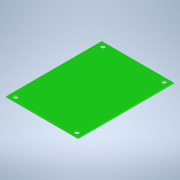
# Autodesk Inventor part: Mock Module PCB
Saved by Autodesk Inventor 2022 (Build 260153000, 153)
## iProperties
Created: 2021-07-19
Part Number: Mock Module PCB
Material: Generic
Document SubType Name: Modeling
Designer: Caleb
Density: 1 g/cm^3
Appearance: Dark Green
Author: Caleb
Autodesk Inventor part; units mm, degrees
(part 1 of 2)
ref_plane "YZ Plane" through (0, 0, 0) normal (1, 0, 0) x (0, 1, 0)
ref_plane "XZ Plane" through (0, 0, 0) normal (0, 1, 0) x (-1, 0, 0)
ref_plane "XY Plane" through (0, 0, 0) normal (0, 0, 1) x (1, 0, 0)
sketch "Sketch1" plane through (0, 0, 0) normal (0, 1, 0) x (-1, 0, 0)
  line L0 (-21.3, 28.25) -> (21.3, 28.25)
  line L1 (21.3, 28.25) -> (21.3, -28.25)
  line L2 (21.3, -28.25) -> (-21.3, -28.25)
  line L3 (-21.3, -28.25) -> (-21.3, 28.25)
  line L4 (-21.3, 28.25) -> (21.3, -28.25) construction
  line L5 (21.3, 28.25) -> (-21.3, -28.25) construction
  point P0 (0, 0)
  dimension "d0" = 42.6
  dimension "d1" = 56.5
  constraints: 12 end point, 2 midpoint, 2 parallel, 1 horizontal, 1 perpendicular
  measures "d0" distance of L0.start L0.end
  measures "d1" distance of L0.end L1.end
extrude "Extrusion1" add sketch "Sketch1" along normal blind 0.5
sketch "Sketch6" plane through (0, 0.5, 0) normal (0, 1, 0) x (1, 0, 0)
  point P0 (0, 0)
  point P1 (-18.05, -25.75)
  point P2 (18.05, -25.75)
  point P3 (18.05, 25.75)
  point P4 (-18.05, 25.75)
  dimension "d33" = 51.5
  dimension "d34" = 36.1
  dimension "d35" = 25.75
  dimension "d36" = 18.05
  constraints: 2 horizontal alignment, 2 vertical alignment
  measures "d33" distance of point (-18.05, -25.75) point (-18.05, 25.75)
  measures "d34" distance of point (18.05, -25.75) point (-18.05, -25.75)
  measures "d35" vertical distance of point (-18.05, -25.75) point (0, 0)
  measures "d36" horizontal distance of point (-18.05, -25.75) point (0, 0)
hole "Hole2" at (-18.05, 0.5, -25.75) at (18.05, 0.5, -25.75) at (18.05, 0.5, 25.75) at (-18.05, 0.5, 25.75) direction (0, -1, 0) diameter 2.2 end through all clearance for "Flat Head Machine Screw" size "M2" standard "Ansi Metric M Profile"
sketch "Sketch7" plane through (0, 0, 0) normal (0, -1, 0) x (1, 0, 0)
  line L0 (-18.3, -24.35) -> (-18.22, -24.35)
  line L1 (-18.22, -24.35) -> (-18.22, -24.05)
  line L2 (-18.22, -24.05) -> (-18.3, -24.05)
  line L3 (-18.3, -24.05) -> (-18.3, -24.35)
  line L4 (-21.3, -28.25) -> (-21.3, 28.25) projected
  line L5 (21.3, -28.25) -> (-21.3, -28.25) projected
  line L6 (-18.175, -24.35) -> (-18.095, -24.35)
  line L7 (-18.095, -24.35) -> (-18.095, -24.05)
  line L8 (-18.095, -24.05) -> (-18.175, -24.05)
  line L9 (-18.175, -24.05) -> (-18.175, -24.35)
  line L10 (-18.05, -24.35) -> (-17.97, -24.35)
  line L11 (-17.97, -24.35) -> (-17.97, -24.05)
  line L12 (-17.97, -24.05) -> (-18.05, -24.05)
  line L13 (-18.05, -24.05) -> (-18.05, -24.35)
  line L14 (-17.925, -24.35) -> (-17.845, -24.35)
  line L15 (-17.845, -24.35) -> (-17.845, -24.05)
  line L16 (-17.845, -24.05) -> (-17.925, -24.05)
  line L17 (-17.925, -24.05) -> (-17.925, -24.35)
  line L18 (-17.8, -24.35) -> (-17.72, -24.35)
  line L19 (-17.72, -24.35) -> (-17.72, -24.05)
  line L20 (-17.72, -24.05) -> (-17.8, -24.05)
  line L21 (-17.8, -24.05) -> (-17.8, -24.35)
  line L22 (-17.675, -24.35) -> (-17.595, -24.35)
  line L23 (-17.595, -24.35) -> (-17.595, -24.05)
  line L24 (-17.595, -24.05) -> (-17.675, -24.05)
  line L25 (-17.675, -24.05) -> (-17.675, -24.35)
  line L26 (-17.55, -24.35) -> (-17.47, -24.35)
  line L27 (-17.47, -24.35) -> (-17.47, -24.05)
  line L28 (-17.47, -24.05) -> (-17.55, -24.05)
  line L29 (-17.55, -24.05) -> (-17.55, -24.35)
  line L30 (-17.425, -24.35) -> (-17.345, -24.35)
  line L31 (-17.345, -24.35) -> (-17.345, -24.05)
  line L32 (-17.345, -24.05) -> (-17.425, -24.05)
  line L33 (-17.425, -24.05) -> (-17.425, -24.35)
  line L34 (-17.3, -24.35) -> (-17.22, -24.35)
  line L35 (-17.22, -24.35) -> (-17.22, -24.05)
  line L36 (-17.22, -24.05) -> (-17.3, -24.05)
  line L37 (-17.3, -24.05) -> (-17.3, -24.35)
  line L38 (-17.175, -24.35) -> (-17.095, -24.35)
  line L39 (-17.095, -24.35) -> (-17.095, -24.05)
  line L40 (-17.095, -24.05) -> (-17.175, -24.05)
  line L41 (-17.175, -24.05) -> (-17.175, -24.35)
  line L42 (-17.05, -24.35) -> (-16.97, -24.35)
  line L43 (-16.97, -24.35) -> (-16.97, -24.05)
  line L44 (-16.97, -24.05) -> (-17.05, -24.05)
  line L45 (-17.05, -24.05) -> (-17.05, -24.35)
  line L46 (-16.925, -24.35) -> (-16.845, -24.35)
  line L47 (-16.845, -24.35) -> (-16.845, -24.05)
  line L48 (-16.845, -24.05) -> (-16.925, -24.05)
  line L49 (-16.925, -24.05) -> (-16.925, -24.35)
  line L50 (-16.8, -24.35) -> (-16.72, -24.35)
  line L51 (-16.72, -24.35) -> (-16.72, -24.05)
  line L52 (-16.72, -24.05) -> (-16.8, -24.05)
  line L53 (-16.8, -24.05) -> (-16.8, -24.35)
  line L54 (-16.675, -24.35) -> (-16.595, -24.35)
  line L55 (-16.595, -24.35) -> (-16.595, -24.05)
  line L56 (-16.595, -24.05) -> (-16.675, -24.05)
  line L57 (-16.675, -24.05) -> (-16.675, -24.35)
  line L58 (-16.55, -24.35) -> (-16.47, -24.35)
  line L59 (-16.47, -24.35) -> (-16.47, -24.05)
  line L60 (-16.47, -24.05) -> (-16.55, -24.05)
  line L61 (-16.55, -24.05) -> (-16.55, -24.35)
  line L62 (-16.425, -24.35) -> (-16.345, -24.35)
  line L63 (-16.345, -24.35) -> (-16.345, -24.05)
  line L64 (-16.345, -24.05) -> (-16.425, -24.05)
  line L65 (-16.425, -24.05) -> (-16.425, -24.35)
  line L66 (-16.3, -24.35) -> (-16.22, -24.35)
  line L67 (-16.22, -24.35) -> (-16.22, -24.05)
  line L68 (-16.22, -24.05) -> (-16.3, -24.05)
  line L69 (-16.3, -24.05) -> (-16.3, -24.35)
  line L70 (-16.175, -24.35) -> (-16.095, -24.35)
  line L71 (-16.095, -24.35) -> (-16.095, -24.05)
  line L72 (-16.095, -24.05) -> (-16.175, -24.05)
  line L73 (-16.175, -24.05) -> (-16.175, -24.35)
  line L74 (-16.05, -24.35) -> (-15.97, -24.35)
  line L75 (-15.97, -24.35) -> (-15.97, -24.05)
  line L76 (-15.97, -24.05) -> (-16.05, -24.05)
  line L77 (-16.05, -24.05) -> (-16.05, -24.35)
  line L78 (-15.925, -24.35) -> (-15.845, -24.35)
  line L79 (-15.845, -24.35) -> (-15.845, -24.05)
  line L80 (-15.845, -24.05) -> (-15.925, -24.05)
  line L81 (-15.925, -24.05) -> (-15.925, -24.35)
  line L82 (-15.8, -24.35) -> (-15.72, -24.35)
  line L83 (-15.72, -24.35) -> (-15.72, -24.05)
  line L84 (-15.72, -24.05) -> (-15.8, -24.05)
  line L85 (-15.8, -24.05) -> (-15.8, -24.35)
  line L86 (-15.675, -24.35) -> (-15.595, -24.35)
  line L87 (-15.595, -24.35) -> (-15.595, -24.05)
  line L88 (-15.595, -24.05) -> (-15.675, -24.05)
  line L89 (-15.675, -24.05) -> (-15.675, -24.35)
  line L90 (-15.55, -24.35) -> (-15.47, -24.35)
  line L91 (-15.47, -24.35) -> (-15.47, -24.05)
  line L92 (-15.47, -24.05) -> (-15.55, -24.05)
  line L93 (-15.55, -24.05) -> (-15.55, -24.35)
  line L94 (-15.425, -24.35) -> (-15.345, -24.35)
  line L95 (-15.345, -24.35) -> (-15.345, -24.05)
  line L96 (-15.345, -24.05) -> (-15.425, -24.05)
  line L97 (-15.425, -24.05) -> (-15.425, -24.35)
  line L98 (-15.3, -24.35) -> (-15.22, -24.35)
  line L99 (-15.22, -24.35) -> (-15.22, -24.05)
  line L100 (-15.22, -24.05) -> (-15.3, -24.05)
  line L101 (-15.3, -24.05) -> (-15.3, -24.35)
  line L102 (-15.175, -24.35) -> (-15.095, -24.35)
  line L103 (-15.095, -24.35) -> (-15.095, -24.05)
  line L104 (-15.095, -24.05) -> (-15.175, -24.05)
  line L105 (-15.175, -24.05) -> (-15.175, -24.35)
  line L106 (-15.05, -24.35) -> (-14.97, -24.35)
  line L107 (-14.97, -24.35) -> (-14.97, -24.05)
  line L108 (-14.97, -24.05) -> (-15.05, -24.05)
  line L109 (-15.05, -24.05) -> (-15.05, -24.35)
  line L110 (-14.925, -24.35) -> (-14.845, -24.35)
  line L111 (-14.845, -24.35) -> (-14.845, -24.05)
  line L112 (-14.845, -24.05) -> (-14.925, -24.05)
  line L113 (-14.925, -24.05) -> (-14.925, -24.35)
  line L114 (-14.8, -24.35) -> (-14.72, -24.35)
  line L115 (-14.72, -24.35) -> (-14.72, -24.05)
  line L116 (-14.72, -24.05) -> (-14.8, -24.05)
  line L117 (-14.8, -24.05) -> (-14.8, -24.35)
  line L118 (-14.675, -24.35) -> (-14.595, -24.35)
  line L119 (-14.595, -24.35) -> (-14.595, -24.05)
  line L120 (-14.595, -24.05) -> (-14.675, -24.05)
  line L121 (-14.675, -24.05) -> (-14.675, -24.35)
  line L122 (-14.55, -24.35) -> (-14.47, -24.35)
  line L123 (-14.47, -24.35) -> (-14.47, -24.05)
  line L124 (-14.47, -24.05) -> (-14.55, -24.05)
  line L125 (-14.55, -24.05) -> (-14.55, -24.35)
  line L126 (-14.425, -24.35) -> (-14.345, -24.35)
  line L127 (-14.345, -24.35) -> (-14.345, -24.05)
  line L128 (-14.345, -24.05) -> (-14.425, -24.05)
  line L129 (-14.425, -24.05) -> (-14.425, -24.35)
  line L130 (-14.3, -24.35) -> (-14.22, -24.35)
  line L131 (-14.22, -24.35) -> (-14.22, -24.05)
  line L132 (-14.22, -24.05) -> (-14.3, -24.05)
  line L133 (-14.3, -24.05) -> (-14.3, -24.35)
  line L134 (-14.175, -24.35) -> (-14.095, -24.35)
  line L135 (-14.095, -24.35) -> (-14.095, -24.05)
  line L136 (-14.095, -24.05) -> (-14.175, -24.05)
  line L137 (-14.175, -24.05) -> (-14.175, -24.35)
  line L138 (-14.05, -24.35) -> (-13.97, -24.35)
  line L139 (-13.97, -24.35) -> (-13.97, -24.05)
  line L140 (-13.97, -24.05) -> (-14.05, -24.05)
  line L141 (-14.05, -24.05) -> (-14.05, -24.35)
  line L142 (-13.925, -24.35) -> (-13.845, -24.35)
  line L143 (-13.845, -24.35) -> (-13.845, -24.05)
  line L144 (-13.845, -24.05) -> (-13.925, -24.05)
  line L145 (-13.925, -24.05) -> (-13.925, -24.35)
  line L146 (-13.8, -24.35) -> (-13.72, -24.35)
  line L147 (-13.72, -24.35) -> (-13.72, -24.05)
  line L148 (-13.72, -24.05) -> (-13.8, -24.05)
  line L149 (-13.8, -24.05) -> (-13.8, -24.35)
  line L150 (-13.675, -24.35) -> (-13.595, -24.35)
  line L151 (-13.595, -24.35) -> (-13.595, -24.05)
  line L152 (-13.595, -24.05) -> (-13.675, -24.05)
  line L153 (-13.675, -24.05) -> (-13.675, -24.35)
  line L154 (-13.55, -24.35) -> (-13.47, -24.35)
  line L155 (-13.47, -24.35) -> (-13.47, -24.05)
  line L156 (-13.47, -24.05) -> (-13.55, -24.05)
  line L157 (-13.55, -24.05) -> (-13.55, -24.35)
  line L158 (-13.425, -24.35) -> (-13.345, -24.35)
  line L159 (-13.345, -24.35) -> (-13.345, -24.05)
  line L160 (-13.345, -24.05) -> (-13.425, -24.05)
  line L161 (-13.425, -24.05) -> (-13.425, -24.35)
  line L162 (-13.3, -24.35) -> (-13.22, -24.35)
  line L163 (-13.22, -24.35) -> (-13.22, -24.05)
  line L164 (-13.22, -24.05) -> (-13.3, -24.05)
  line L165 (-13.3, -24.05) -> (-13.3, -24.35)
  line L166 (-13.175, -24.35) -> (-13.095, -24.35)
  line L167 (-13.095, -24.35) -> (-13.095, -24.05)
  line L168 (-13.095, -24.05) -> (-13.175, -24.05)
  line L169 (-13.175, -24.05) -> (-13.175, -24.35)
  line L170 (-13.05, -24.35) -> (-12.97, -24.35)
  line L171 (-12.97, -24.35) -> (-12.97, -24.05)
  line L172 (-12.97, -24.05) -> (-13.05, -24.05)
  line L173 (-13.05, -24.05) -> (-13.05, -24.35)
  line L174 (-12.925, -24.35) -> (-12.845, -24.35)
  line L175 (-12.845, -24.35) -> (-12.845, -24.05)
  line L176 (-12.845, -24.05) -> (-12.925, -24.05)
  line L177 (-12.925, -24.05) -> (-12.925, -24.35)
  line L178 (-12.8, -24.35) -> (-12.72, -24.35)
  line L179 (-12.72, -24.35) -> (-12.72, -24.05)
  line L180 (-12.72, -24.05) -> (-12.8, -24.05)
  line L181 (-12.8, -24.05) -> (-12.8, -24.35)
  line L182 (-12.675, -24.35) -> (-12.595, -24.35)
  line L183 (-12.595, -24.35) -> (-12.595, -24.05)
  line L184 (-12.595, -24.05) -> (-12.675, -24.05)
  line L185 (-12.675, -24.05) -> (-12.675, -24.35)
  line L186 (-12.55, -24.35) -> (-12.47, -24.35)
  line L187 (-12.47, -24.35) -> (-12.47, -24.05)
  line L188 (-12.47, -24.05) -> (-12.55, -24.05)
  line L189 (-12.55, -24.05) -> (-12.55, -24.35)
  line L190 (-12.425, -24.35) -> (-12.345, -24.35)
  line L191 (-12.345, -24.35) -> (-12.345, -24.05)
  line L192 (-12.345, -24.05) -> (-12.425, -24.05)
  line L193 (-12.425, -24.05) -> (-12.425, -24.35)
  line L194 (-12.3, -24.35) -> (-12.22, -24.35)
  line L195 (-12.22, -24.35) -> (-12.22, -24.05)
  line L196 (-12.22, -24.05) -> (-12.3, -24.05)
  line L197 (-12.3, -24.05) -> (-12.3, -24.35)
  line L198 (-12.175, -24.35) -> (-12.095, -24.35)
  line L199 (-12.095, -24.35) -> (-12.095, -24.05)
  line L200 (-12.095, -24.05) -> (-12.175, -24.05)
  line L201 (-12.175, -24.05) -> (-12.175, -24.35)
  line L202 (-12.05, -24.35) -> (-11.97, -24.35)
  line L203 (-11.97, -24.35) -> (-11.97, -24.05)
  line L204 (-11.97, -24.05) -> (-12.05, -24.05)
  line L205 (-12.05, -24.05) -> (-12.05, -24.35)
  line L206 (-11.925, -24.35) -> (-11.845, -24.35)
  line L207 (-11.845, -24.35) -> (-11.845, -24.05)
  line L208 (-11.845, -24.05) -> (-11.925, -24.05)
  line L209 (-11.925, -24.05) -> (-11.925, -24.35)
  line L210 (-11.8, -24.35) -> (-11.72, -24.35)
  line L211 (-11.72, -24.35) -> (-11.72, -24.05)
  line L212 (-11.72, -24.05) -> (-11.8, -24.05)
  line L213 (-11.8, -24.05) -> (-11.8, -24.35)
  line L214 (-11.675, -24.35) -> (-11.595, -24.35)
  line L215 (-11.595, -24.35) -> (-11.595, -24.05)
  line L216 (-11.595, -24.05) -> (-11.675, -24.05)
  line L217 (-11.675, -24.05) -> (-11.675, -24.35)
  line L218 (-11.55, -24.35) -> (-11.47, -24.35)
  line L219 (-11.47, -24.35) -> (-11.47, -24.05)
  line L220 (-11.47, -24.05) -> (-11.55, -24.05)
  line L221 (-11.55, -24.05) -> (-11.55, -24.35)
  line L222 (-11.425, -24.35) -> (-11.345, -24.35)
  line L223 (-11.345, -24.35) -> (-11.345, -24.05)
  line L224 (-11.345, -24.05) -> (-11.425, -24.05)
  line L225 (-11.425, -24.05) -> (-11.425, -24.35)
  line L226 (-11.3, -24.35) -> (-11.22, -24.35)
  line L227 (-11.22, -24.35) -> (-11.22, -24.05)
  line L228 (-11.22, -24.05) -> (-11.3, -24.05)
  line L229 (-11.3, -24.05) -> (-11.3, -24.35)
  line L230 (-11.175, -24.35) -> (-11.095, -24.35)
  line L231 (-11.095, -24.35) -> (-11.095, -24.05)
  line L232 (-11.095, -24.05) -> (-11.175, -24.05)
  line L233 (-11.175, -24.05) -> (-11.175, -24.35)
  line L234 (-11.05, -24.35) -> (-10.97, -24.35)
  line L235 (-10.97, -24.35) -> (-10.97, -24.05)
  line L236 (-10.97, -24.05) -> (-11.05, -24.05)
  line L237 (-11.05, -24.05) -> (-11.05, -24.35)
  line L238 (-10.925, -24.35) -> (-10.845, -24.35)
  line L239 (-10.845, -24.35) -> (-10.845, -24.05)
  line L240 (-10.845, -24.05) -> (-10.925, -24.05)
  line L241 (-10.925, -24.05) -> (-10.925, -24.35)
  line L242 (-10.8, -24.35) -> (-10.72, -24.35)
  line L243 (-10.72, -24.35) -> (-10.72, -24.05)
  line L244 (-10.72, -24.05) -> (-10.8, -24.05)
  line L245 (-10.8, -24.05) -> (-10.8, -24.35)
  line L246 (-10.675, -24.35) -> (-10.595, -24.35)
  line L247 (-10.595, -24.35) -> (-10.595, -24.05)
  line L248 (-10.595, -24.05) -> (-10.675, -24.05)
  line L249 (-10.675, -24.05) -> (-10.675, -24.35)
  line L250 (-10.55, -24.35) -> (-10.47, -24.35)
  line L251 (-10.47, -24.35) -> (-10.47, -24.05)
  line L252 (-10.47, -24.05) -> (-10.55, -24.05)
  line L253 (-10.55, -24.05) -> (-10.55, -24.35)
  line L254 (-10.425, -24.35) -> (-10.345, -24.35)
  line L255 (-10.345, -24.35) -> (-10.345, -24.05)
  line L256 (-10.345, -24.05) -> (-10.425, -24.05)
  line L257 (-10.425, -24.05) -> (-10.425, -24.35)
  line L258 (-10.3, -24.35) -> (-10.22, -24.35)
  line L259 (-10.22, -24.35) -> (-10.22, -24.05)
  line L260 (-10.22, -24.05) -> (-10.3, -24.05)
  line L261 (-10.3, -24.05) -> (-10.3, -24.35)
  line L262 (-10.175, -24.35) -> (-10.095, -24.35)
  line L263 (-10.095, -24.35) -> (-10.095, -24.05)
  line L264 (-10.095, -24.05) -> (-10.175, -24.05)
  line L265 (-10.175, -24.05) -> (-10.175, -24.35)
  line L266 (-10.05, -24.35) -> (-9.97, -24.35)
  line L267 (-9.97, -24.35) -> (-9.97, -24.05)
  line L268 (-9.97, -24.05) -> (-10.05, -24.05)
  line L269 (-10.05, -24.05) -> (-10.05, -24.35)
  line L270 (-9.925, -24.35) -> (-9.845, -24.35)
  line L271 (-9.845, -24.35) -> (-9.845, -24.05)
  line L272 (-9.845, -24.05) -> (-9.925, -24.05)
  line L273 (-9.925, -24.05) -> (-9.925, -24.35)
  line L274 (-9.8, -24.35) -> (-9.72, -24.35)
  line L275 (-9.72, -24.35) -> (-9.72, -24.05)
  line L276 (-9.72, -24.05) -> (-9.8, -24.05)
  line L277 (-9.8, -24.05) -> (-9.8, -24.35)
  line L278 (-9.675, -24.35) -> (-9.595, -24.35)
  line L279 (-9.595, -24.35) -> (-9.595, -24.05)
  line L280 (-9.595, -24.05) -> (-9.675, -24.05)
  line L281 (-9.675, -24.05) -> (-9.675, -24.35)
  line L282 (-9.55, -24.35) -> (-9.47, -24.35)
  line L283 (-9.47, -24.35) -> (-9.47, -24.05)
  line L284 (-9.47, -24.05) -> (-9.55, -24.05)
  line L285 (-9.55, -24.05) -> (-9.55, -24.35)
  line L286 (-9.425, -24.35) -> (-9.345, -24.35)
  line L287 (-9.345, -24.35) -> (-9.345, -24.05)
  line L288 (-9.345, -24.05) -> (-9.425, -24.05)
  line L289 (-9.425, -24.05) -> (-9.425, -24.35)
  line L290 (-9.3, -24.35) -> (-9.22, -24.35)
  line L291 (-9.22, -24.35) -> (-9.22, -24.05)
  line L292 (-9.22, -24.05) -> (-9.3, -24.05)
  line L293 (-9.3, -24.05) -> (-9.3, -24.35)
  line L294 (-9.175, -24.35) -> (-9.095, -24.35)
  line L295 (-9.095, -24.35) -> (-9.095, -24.05)
  line L296 (-9.095, -24.05) -> (-9.175, -24.05)
  line L297 (-9.175, -24.05) -> (-9.175, -24.35)
  line L298 (-9.05, -24.35) -> (-8.97, -24.35)
  line L299 (-8.97, -24.35) -> (-8.97, -24.05)
  line L300 (-8.97, -24.05) -> (-9.05, -24.05)
  line L301 (-9.05, -24.05) -> (-9.05, -24.35)
  line L302 (-8.925, -24.35) -> (-8.845, -24.35)
  line L303 (-8.845, -24.35) -> (-8.845, -24.05)
  line L304 (-8.845, -24.05) -> (-8.925, -24.05)
  line L305 (-8.925, -24.05) -> (-8.925, -24.35)
  line L306 (-8.8, -24.35) -> (-8.72, -24.35)
  line L307 (-8.72, -24.35) -> (-8.72, -24.05)
  line L308 (-8.72, -24.05) -> (-8.8, -24.05)
  line L309 (-8.8, -24.05) -> (-8.8, -24.35)
  line L310 (-8.675, -24.35) -> (-8.595, -24.35)
  line L311 (-8.595, -24.35) -> (-8.595, -24.05)
  line L312 (-8.595, -24.05) -> (-8.675, -24.05)
  line L313 (-8.675, -24.05) -> (-8.675, -24.35)
  line L314 (-8.55, -24.35) -> (-8.47, -24.35)
  line L315 (-8.47, -24.35) -> (-8.47, -24.05)
  line L316 (-8.47, -24.05) -> (-8.55, -24.05)
  line L317 (-8.55, -24.05) -> (-8.55, -24.35)
  line L318 (-8.425, -24.35) -> (-8.345, -24.35)
  line L319 (-8.345, -24.35) -> (-8.345, -24.05)
  line L320 (-8.345, -24.05) -> (-8.425, -24.05)
  line L321 (-8.425, -24.05) -> (-8.425, -24.35)
  line L322 (-8.3, -24.35) -> (-8.22, -24.35)
  line L323 (-8.22, -24.35) -> (-8.22, -24.05)
  line L324 (-8.22, -24.05) -> (-8.3, -24.05)
  line L325 (-8.3, -24.05) -> (-8.3, -24.35)
  line L326 (-8.175, -24.35) -> (-8.095, -24.35)
  line L327 (-8.095, -24.35) -> (-8.095, -24.05)
  line L328 (-8.095, -24.05) -> (-8.175, -24.05)
  line L329 (-8.175, -24.05) -> (-8.175, -24.35)
  line L330 (-8.05, -24.35) -> (-7.97, -24.35)
  line L331 (-7.97, -24.35) -> (-7.97, -24.05)
  line L332 (-7.97, -24.05) -> (-8.05, -24.05)
  line L333 (-8.05, -24.05) -> (-8.05, -24.35)
  line L334 (-7.925, -24.35) -> (-7.845, -24.35)
  line L335 (-7.845, -24.35) -> (-7.845, -24.05)
  line L336 (-7.845, -24.05) -> (-7.925, -24.05)
  line L337 (-7.925, -24.05) -> (-7.925, -24.35)
  line L338 (-7.8, -24.35) -> (-7.72, -24.35)
  line L339 (-7.72, -24.35) -> (-7.72, -24.05)
  line L340 (-7.72, -24.05) -> (-7.8, -24.05)
  line L341 (-7.8, -24.05) -> (-7.8, -24.35)
  line L342 (-7.675, -24.35) -> (-7.595, -24.35)
  line L343 (-7.595, -24.35) -> (-7.595, -24.05)
  line L344 (-7.595, -24.05) -> (-7.675, -24.05)
  line L345 (-7.675, -24.05) -> (-7.675, -24.35)
  line L346 (-7.55, -24.35) -> (-7.47, -24.35)
  line L347 (-7.47, -24.35) -> (-7.47, -24.05)
  line L348 (-7.47, -24.05) -> (-7.55, -24.05)
  line L349 (-7.55, -24.05) -> (-7.55, -24.35)
  line L350 (-7.425, -24.35) -> (-7.345, -24.35)
  line L351 (-7.345, -24.35) -> (-7.345, -24.05)
  line L352 (-7.345, -24.05) -> (-7.425, -24.05)
  line L353 (-7.425, -24.05) -> (-7.425, -24.35)
  line L354 (-7.3, -24.35) -> (-7.22, -24.35)
  line L355 (-7.22, -24.35) -> (-7.22, -24.05)
  line L356 (-7.22, -24.05) -> (-7.3, -24.05)
  line L357 (-7.3, -24.05) -> (-7.3, -24.35)
  line L358 (-7.175, -24.35) -> (-7.095, -24.35)
  line L359 (-7.095, -24.35) -> (-7.095, -24.05)
  line L360 (-7.095, -24.05) -> (-7.175, -24.05)
  line L361 (-7.175, -24.05) -> (-7.175, -24.35)
  line L362 (-7.05, -24.35) -> (-6.97, -24.35)
  line L363 (-6.97, -24.35) -> (-6.97, -24.05)
  line L364 (-6.97, -24.05) -> (-7.05, -24.05)
  line L365 (-7.05, -24.05) -> (-7.05, -24.35)
  line L366 (-6.925, -24.35) -> (-6.845, -24.35)
  line L367 (-6.845, -24.35) -> (-6.845, -24.05)
  line L368 (-6.845, -24.05) -> (-6.925, -24.05)
  line L369 (-6.925, -24.05) -> (-6.925, -24.35)
  line L370 (-6.8, -24.35) -> (-6.72, -24.35)
  line L371 (-6.72, -24.35) -> (-6.72, -24.05)
  line L372 (-6.72, -24.05) -> (-6.8, -24.05)
  line L373 (-6.8, -24.05) -> (-6.8, -24.35)
  line L374 (-6.675, -24.35) -> (-6.595, -24.35)
  line L375 (-6.595, -24.35) -> (-6.595, -24.05)
  line L376 (-6.595, -24.05) -> (-6.675, -24.05)
  line L377 (-6.675, -24.05) -> (-6.675, -24.35)
  line L378 (-6.55, -24.35) -> (-6.47, -24.35)
  line L379 (-6.47, -24.35) -> (-6.47, -24.05)
  line L380 (-6.47, -24.05) -> (-6.55, -24.05)
  line L381 (-6.55, -24.05) -> (-6.55, -24.35)
  line L382 (-6.425, -24.35) -> (-6.345, -24.35)
  line L383 (-6.345, -24.35) -> (-6.345, -24.05)
  line L384 (-6.345, -24.05) -> (-6.425, -24.05)
  line L385 (-6.425, -24.05) -> (-6.425, -24.35)
  line L386 (-6.3, -24.35) -> (-6.22, -24.35)
  line L387 (-6.22, -24.35) -> (-6.22, -24.05)
  line L388 (-6.22, -24.05) -> (-6.3, -24.05)
  line L389 (-6.3, -24.05) -> (-6.3, -24.35)
  line L390 (-6.175, -24.35) -> (-6.095, -24.35)
  line L391 (-6.095, -24.35) -> (-6.095, -24.05)
  line L392 (-6.095, -24.05) -> (-6.175, -24.05)
  line L393 (-6.175, -24.05) -> (-6.175, -24.35)
  line L394 (-6.05, -24.35) -> (-5.97, -24.35)
  line L395 (-5.97, -24.35) -> (-5.97, -24.05)
  line L396 (-5.97, -24.05) -> (-6.05, -24.05)
  line L397 (-6.05, -24.05) -> (-6.05, -24.35)
  line L398 (-5.925, -24.35) -> (-5.845, -24.35)
  line L399 (-5.845, -24.35) -> (-5.845, -24.05)
  line L400 (-5.845, -24.05) -> (-5.925, -24.05)
  line L401 (-5.925, -24.05) -> (-5.925, -24.35)
  line L402 (-5.8, -24.35) -> (-5.72, -24.35)
  line L403 (-5.72, -24.35) -> (-5.72, -24.05)
  line L404 (-5.72, -24.05) -> (-5.8, -24.05)
  line L405 (-5.8, -24.05) -> (-5.8, -24.35)
  line L406 (-5.675, -24.35) -> (-5.595, -24.35)
  line L407 (-5.595, -24.35) -> (-5.595, -24.05)
  line L408 (-5.595, -24.05) -> (-5.675, -24.05)
  line L409 (-5.675, -24.05) -> (-5.675, -24.35)
  line L410 (-5.55, -24.35) -> (-5.47, -24.35)
  line L411 (-5.47, -24.35) -> (-5.47, -24.05)
  line L412 (-5.47, -24.05) -> (-5.55, -24.05)
  line L413 (-5.55, -24.05) -> (-5.55, -24.35)
  line L414 (-5.425, -24.35) -> (-5.345, -24.35)
  line L415 (-5.345, -24.35) -> (-5.345, -24.05)
  line L416 (-5.345, -24.05) -> (-5.425, -24.05)
  line L417 (-5.425, -24.05) -> (-5.425, -24.35)
  line L418 (-5.3, -24.35) -> (-5.22, -24.35)
  line L419 (-5.22, -24.35) -> (-5.22, -24.05)
  line L420 (-5.22, -24.05) -> (-5.3, -24.05)
  line L421 (-5.3, -24.05) -> (-5.3, -24.35)
  line L422 (-5.175, -24.35) -> (-5.095, -24.35)
  line L423 (-5.095, -24.35) -> (-5.095, -24.05)
  line L424 (-5.095, -24.05) -> (-5.175, -24.05)
  line L425 (-5.175, -24.05) -> (-5.175, -24.35)
  line L426 (-5.05, -24.35) -> (-4.97, -24.35)
  line L427 (-4.97, -24.35) -> (-4.97, -24.05)
  line L428 (-4.97, -24.05) -> (-5.05, -24.05)
  line L429 (-5.05, -24.05) -> (-5.05, -24.35)
  line L430 (-4.925, -24.35) -> (-4.845, -24.35)
  line L431 (-4.845, -24.35) -> (-4.845, -24.05)
  line L432 (-4.845, -24.05) -> (-4.925, -24.05)
  line L433 (-4.925, -24.05) -> (-4.925, -24.35)
  line L434 (-4.8, -24.35) -> (-4.72, -24.35)
  line L435 (-4.72, -24.35) -> (-4.72, -24.05)
  line L436 (-4.72, -24.05) -> (-4.8, -24.05)
  line L437 (-4.8, -24.05) -> (-4.8, -24.35)
  line L438 (-4.675, -24.35) -> (-4.595, -24.35)
  line L439 (-4.595, -24.35) -> (-4.595, -24.05)
  line L440 (-4.595, -24.05) -> (-4.675, -24.05)
  line L441 (-4.675, -24.05) -> (-4.675, -24.35)
  line L442 (-4.55, -24.35) -> (-4.47, -24.35)
  line L443 (-4.47, -24.35) -> (-4.47, -24.05)
  line L444 (-4.47, -24.05) -> (-4.55, -24.05)
  line L445 (-4.55, -24.05) -> (-4.55, -24.35)
  line L446 (-4.425, -24.35) -> (-4.345, -24.35)
  line L447 (-4.345, -24.35) -> (-4.345, -24.05)
  line L448 (-4.345, -24.05) -> (-4.425, -24.05)
  line L449 (-4.425, -24.05) -> (-4.425, -24.35)
  line L450 (-4.3, -24.35) -> (-4.22, -24.35)
  line L451 (-4.22, -24.35) -> (-4.22, -24.05)
  line L452 (-4.22, -24.05) -> (-4.3, -24.05)
  line L453 (-4.3, -24.05) -> (-4.3, -24.35)
  line L454 (-4.175, -24.35) -> (-4.095, -24.35)
  line L455 (-4.095, -24.35) -> (-4.095, -24.05)
  line L456 (-4.095, -24.05) -> (-4.175, -24.05)
  line L457 (-4.175, -24.05) -> (-4.175, -24.35)
  line L458 (-4.05, -24.35) -> (-3.97, -24.35)
  line L459 (-3.97, -24.35) -> (-3.97, -24.05)
  line L460 (-3.97, -24.05) -> (-4.05, -24.05)
  line L461 (-4.05, -24.05) -> (-4.05, -24.35)
  line L462 (-3.925, -24.35) -> (-3.845, -24.35)
  line L463 (-3.845, -24.35) -> (-3.845, -24.05)
  line L464 (-3.845, -24.05) -> (-3.925, -24.05)
  line L465 (-3.925, -24.05) -> (-3.925, -24.35)
  line L466 (-3.8, -24.35) -> (-3.72, -24.35)
  line L467 (-3.72, -24.35) -> (-3.72, -24.05)
  line L468 (-3.72, -24.05) -> (-3.8, -24.05)
  line L469 (-3.8, -24.05) -> (-3.8, -24.35)
  line L470 (-3.675, -24.35) -> (-3.595, -24.35)
  line L471 (-3.595, -24.35) -> (-3.595, -24.05)
  line L472 (-3.595, -24.05) -> (-3.675, -24.05)
  line L473 (-3.675, -24.05) -> (-3.675, -24.35)
  line L474 (-3.55, -24.35) -> (-3.47, -24.35)
  line L475 (-3.47, -24.35) -> (-3.47, -24.05)
  line L476 (-3.47, -24.05) -> (-3.55, -24.05)
  line L477 (-3.55, -24.05) -> (-3.55, -24.35)
  line L478 (-3.425, -24.35) -> (-3.345, -24.35)
  line L479 (-3.345, -24.35) -> (-3.345, -24.05)
  line L480 (-3.345, -24.05) -> (-3.425, -24.05)
  line L481 (-3.425, -24.05) -> (-3.425, -24.35)
  line L482 (-3.3, -24.35) -> (-3.22, -24.35)
  line L483 (-3.22, -24.35) -> (-3.22, -24.05)
  line L484 (-3.22, -24.05) -> (-3.3, -24.05)
  line L485 (-3.3, -24.05) -> (-3.3, -24.35)
  line L486 (-3.175, -24.35) -> (-3.095, -24.35)
  line L487 (-3.095, -24.35) -> (-3.095, -24.05)
  line L488 (-3.095, -24.05) -> (-3.175, -24.05)
  line L489 (-3.175, -24.05) -> (-3.175, -24.35)
  line L490 (-3.05, -24.35) -> (-2.97, -24.35)
  line L491 (-2.97, -24.35) -> (-2.97, -24.05)
  line L492 (-2.97, -24.05) -> (-3.05, -24.05)
  line L493 (-3.05, -24.05) -> (-3.05, -24.35)
  line L494 (-2.925, -24.35) -> (-2.845, -24.35)
  line L495 (-2.845, -24.35) -> (-2.845, -24.05)
  line L496 (-2.845, -24.05) -> (-2.925, -24.05)
  line L497 (-2.925, -24.05) -> (-2.925, -24.35)
  line L498 (-2.8, -24.35) -> (-2.72, -24.35)
  line L499 (-2.72, -24.35) -> (-2.72, -24.05)
  line L500 (-2.72, -24.05) -> (-2.8, -24.05)
  line L501 (-2.8, -24.05) -> (-2.8, -24.35)
  line L502 (-2.675, -24.35) -> (-2.595, -24.35)
  line L503 (-2.595, -24.35) -> (-2.595, -24.05)
  line L504 (-2.595, -24.05) -> (-2.675, -24.05)
  line L505 (-2.675, -24.05) -> (-2.675, -24.35)
  line L506 (-2.55, -24.35) -> (-2.47, -24.35)
  line L507 (-2.47, -24.35) -> (-2.47, -24.05)
  line L508 (-2.47, -24.05) -> (-2.55, -24.05)
  line L509 (-2.55, -24.05) -> (-2.55, -24.35)
  line L510 (-2.425, -24.35) -> (-2.345, -24.35)
  line L511 (-2.345, -24.35) -> (-2.345, -24.05)
  line L512 (-2.345, -24.05) -> (-2.425, -24.05)
  line L513 (-2.425, -24.05) -> (-2.425, -24.35)
  line L514 (-2.3, -24.35) -> (-2.22, -24.35)
  line L515 (-2.22, -24.35) -> (-2.22, -24.05)
  line L516 (-2.22, -24.05) -> (-2.3, -24.05)
  line L517 (-2.3, -24.05) -> (-2.3, -24.35)
  line L518 (-2.175, -24.35) -> (-2.095, -24.35)
  line L519 (-2.095, -24.35) -> (-2.095, -24.05)
  line L520 (-2.095, -24.05) -> (-2.175, -24.05)
  line L521 (-2.175, -24.05) -> (-2.175, -24.35)
  line L522 (-2.05, -24.35) -> (-1.97, -24.35)
  line L523 (-1.97, -24.35) -> (-1.97, -24.05)
  line L524 (-1.97, -24.05) -> (-2.05, -24.05)
  line L525 (-2.05, -24.05) -> (-2.05, -24.35)
  line L526 (-1.925, -24.35) -> (-1.845, -24.35)
  line L527 (-1.845, -24.35) -> (-1.845, -24.05)
  line L528 (-1.845, -24.05) -> (-1.925, -24.05)
  line L529 (-1.925, -24.05) -> (-1.925, -24.35)
  line L530 (-1.8, -24.35) -> (-1.72, -24.35)
  line L531 (-1.72, -24.35) -> (-1.72, -24.05)
  line L532 (-1.72, -24.05) -> (-1.8, -24.05)
  line L533 (-1.8, -24.05) -> (-1.8, -24.35)
  line L534 (-1.675, -24.35) -> (-1.595, -24.35)
  line L535 (-1.595, -24.35) -> (-1.595, -24.05)
  line L536 (-1.595, -24.05) -> (-1.675, -24.05)
  line L537 (-1.675, -24.05) -> (-1.675, -24.35)
  line L538 (-1.55, -24.35) -> (-1.47, -24.35)
  line L539 (-1.47, -24.35) -> (-1.47, -24.05)
  line L540 (-1.47, -24.05) -> (-1.55, -24.05)
  line L541 (-1.55, -24.05) -> (-1.55, -24.35)
  line L542 (-1.425, -24.35) -> (-1.345, -24.35)
  line L543 (-1.345, -24.35) -> (-1.345, -24.05)
  line L544 (-1.345, -24.05) -> (-1.425, -24.05)
  line L545 (-1.425, -24.05) -> (-1.425, -24.35)
  line L546 (-1.3, -24.35) -> (-1.22, -24.35)
  line L547 (-1.22, -24.35) -> (-1.22, -24.05)
  line L548 (-1.22, -24.05) -> (-1.3, -24.05)
  line L549 (-1.3, -24.05) -> (-1.3, -24.35)
  line L550 (-1.175, -24.35) -> (-1.095, -24.35)
  line L551 (-1.095, -24.35) -> (-1.095, -24.05)
  line L552 (-1.095, -24.05) -> (-1.175, -24.05)
  line L553 (-1.175, -24.05) -> (-1.175, -24.35)
  line L554 (-1.05, -24.35) -> (-0.97, -24.35)
  line L555 (-0.97, -24.35) -> (-0.97, -24.05)
  line L556 (-0.97, -24.05) -> (-1.05, -24.05)
  line L557 (-1.05, -24.05) -> (-1.05, -24.35)
  line L558 (-0.925, -24.35) -> (-0.845, -24.35)
  line L559 (-0.845, -24.35) -> (-0.845, -24.05)
  line L560 (-0.845, -24.05) -> (-0.925, -24.05)
  line L561 (-0.925, -24.05) -> (-0.925, -24.35)
  line L562 (-0.8, -24.35) -> (-0.72, -24.35)
  line L563 (-0.72, -24.35) -> (-0.72, -24.05)
  line L564 (-0.72, -24.05) -> (-0.8, -24.05)
  line L565 (-0.8, -24.05) -> (-0.8, -24.35)
  line L566 (-0.675, -24.35) -> (-0.595, -24.35)
  line L567 (-0.595, -24.35) -> (-0.595, -24.05)
  line L568 (-0.595, -24.05) -> (-0.675, -24.05)
  line L569 (-0.675, -24.05) -> (-0.675, -24.35)
  point P0 (0, 0)
  dimension "d44" = 0.08
  dimension "d45" = 0.3
  dimension "d46" = 3
  dimension "d47" = 3.9
  dimension "d50" = 0.125
  constraints: 1136 end point, 2 horizontal, 2 parallel, 1 perpendicular, 1128 other
  measures "d44" distance of L1.end L2.end
  measures "d45" distance of L2.end L0.start
  measures "d46" distance between parallel lines of L4 L3
  measures "d47" distance between parallel lines of L5 L0
  measures "d50" distance of L0.start L6.start
extrude "Extrusion3" add sketch "Sketch7" along normal blind 0.05
sketch "Sketch8" plane through (0, 0, 0) normal (0, -1, 0) x (1, 0, 0)
  line L0 (18.3, 24.35) -> (18.2238, 24.35)
  line L1 (18.2238, 24.35) -> (18.2238, 24.05)
  line L2 (18.2238, 24.05) -> (18.3, 24.05)
  line L3 (18.3, 24.05) -> (18.3, 24.35)
  line L4 (21.3, 28.25) -> (21.3, -28.25) projected
  line L5 (-21.3, 28.25) -> (21.3, 28.25) projected
  line L6 (18.05, 24.35) -> (17.9738, 24.35)
  line L7 (17.9738, 24.35) -> (17.9738, 24.05)
  line L8 (17.9738, 24.05) -> (18.05, 24.05)
  line L9 (18.05, 24.05) -> (18.05, 24.35)
  line L10 (17.8, 24.35) -> (17.7238, 24.35)
  line L11 (17.7238, 24.35) -> (17.7238, 24.05)
  line L12 (17.7238, 24.05) -> (17.8, 24.05)
  line L13 (17.8, 24.05) -> (17.8, 24.35)
  line L14 (17.55, 24.35) -> (17.4738, 24.35)
  line L15 (17.4738, 24.35) -> (17.4738, 24.05)
  line L16 (17.4738, 24.05) -> (17.55, 24.05)
  line L17 (17.55, 24.05) -> (17.55, 24.35)
  line L18 (17.3, 24.35) -> (17.2238, 24.35)
  line L19 (17.2238, 24.35) -> (17.2238, 24.05)
  line L20 (17.2238, 24.05) -> (17.3, 24.05)
  line L21 (17.3, 24.05) -> (17.3, 24.35)
  line L22 (17.05, 24.35) -> (16.9738, 24.35)
  line L23 (16.9738, 24.35) -> (16.9738, 24.05)
  line L24 (16.9738, 24.05) -> (17.05, 24.05)
  line L25 (17.05, 24.05) -> (17.05, 24.35)
  line L26 (16.8, 24.35) -> (16.7238, 24.35)
  line L27 (16.7238, 24.35) -> (16.7238, 24.05)
  line L28 (16.7238, 24.05) -> (16.8, 24.05)
  line L29 (16.8, 24.05) -> (16.8, 24.35)
  line L30 (16.55, 24.35) -> (16.4738, 24.35)
  line L31 (16.4738, 24.35) -> (16.4738, 24.05)
  line L32 (16.4738, 24.05) -> (16.55, 24.05)
  line L33 (16.55, 24.05) -> (16.55, 24.35)
  line L34 (16.3, 24.35) -> (16.2238, 24.35)
  line L35 (16.2238, 24.35) -> (16.2238, 24.05)
  line L36 (16.2238, 24.05) -> (16.3, 24.05)
  line L37 (16.3, 24.05) -> (16.3, 24.35)
  line L38 (16.05, 24.35) -> (15.9738, 24.35)
  line L39 (15.9738, 24.35) -> (15.9738, 24.05)
  line L40 (15.9738, 24.05) -> (16.05, 24.05)
  line L41 (16.05, 24.05) -> (16.05, 24.35)
  line L42 (15.8, 24.35) -> (15.7238, 24.35)
  line L43 (15.7238, 24.35) -> (15.7238, 24.05)
  line L44 (15.7238, 24.05) -> (15.8, 24.05)
  line L45 (15.8, 24.05) -> (15.8, 24.35)
  line L46 (15.55, 24.35) -> (15.4738, 24.35)
  line L47 (15.4738, 24.35) -> (15.4738, 24.05)
  line L48 (15.4738, 24.05) -> (15.55, 24.05)
  line L49 (15.55, 24.05) -> (15.55, 24.35)
  line L50 (15.3, 24.35) -> (15.2238, 24.35)
  line L51 (15.2238, 24.35) -> (15.2238, 24.05)
  line L52 (15.2238, 24.05) -> (15.3, 24.05)
  line L53 (15.3, 24.05) -> (15.3, 24.35)
  line L54 (15.05, 24.35) -> (14.9738, 24.35)
  line L55 (14.9738, 24.35) -> (14.9738, 24.05)
  line L56 (14.9738, 24.05) -> (15.05, 24.05)
  line L57 (15.05, 24.05) -> (15.05, 24.35)
  line L58 (14.8, 24.35) -> (14.7238, 24.35)
  line L59 (14.7238, 24.35) -> (14.7238, 24.05)
  line L60 (14.7238, 24.05) -> (14.8, 24.05)
  line L61 (14.8, 24.05) -> (14.8, 24.35)
  line L62 (14.55, 24.35) -> (14.4738, 24.35)
  line L63 (14.4738, 24.35) -> (14.4738, 24.05)
  line L64 (14.4738, 24.05) -> (14.55, 24.05)
  line L65 (14.55, 24.05) -> (14.55, 24.35)
  line L66 (14.3, 24.35) -> (14.2238, 24.35)
  line L67 (14.2238, 24.35) -> (14.2238, 24.05)
  line L68 (14.2238, 24.05) -> (14.3, 24.05)
  line L69 (14.3, 24.05) -> (14.3, 24.35)
  line L70 (14.05, 24.35) -> (13.9738, 24.35)
  line L71 (13.9738, 24.35) -> (13.9738, 24.05)
  line L72 (13.9738, 24.05) -> (14.05, 24.05)
  line L73 (14.05, 24.05) -> (14.05, 24.35)
  line L74 (13.8, 24.35) -> (13.7238, 24.35)
  line L75 (13.7238, 24.35) -> (13.7238, 24.05)
  line L76 (13.7238, 24.05) -> (13.8, 24.05)
  line L77 (13.8, 24.05) -> (13.8, 24.35)
  line L78 (13.55, 24.35) -> (13.4738, 24.35)
  line L79 (13.4738, 24.35) -> (13.4738, 24.05)
  line L80 (13.4738, 24.05) -> (13.55, 24.05)
  line L81 (13.55, 24.05) -> (13.55, 24.35)
  line L82 (13.3, 24.35) -> (13.2238, 24.35)
  line L83 (13.2238, 24.35) -> (13.2238, 24.05)
  line L84 (13.2238, 24.05) -> (13.3, 24.05)
  line L85 (13.3, 24.05) -> (13.3, 24.35)
  line L86 (13.05, 24.35) -> (12.9738, 24.35)
  line L87 (12.9738, 24.35) -> (12.9738, 24.05)
  line L88 (12.9738, 24.05) -> (13.05, 24.05)
  line L89 (13.05, 24.05) -> (13.05, 24.35)
  line L90 (12.8, 24.35) -> (12.7238, 24.35)
  line L91 (12.7238, 24.35) -> (12.7238, 24.05)
  line L92 (12.7238, 24.05) -> (12.8, 24.05)
  line L93 (12.8, 24.05) -> (12.8, 24.35)
  line L94 (12.55, 24.35) -> (12.4738, 24.35)
  line L95 (12.4738, 24.35) -> (12.4738, 24.05)
  line L96 (12.4738, 24.05) -> (12.55, 24.05)
  line L97 (12.55, 24.05) -> (12.55, 24.35)
  line L98 (12.3, 24.35) -> (12.2238, 24.35)
  line L99 (12.2238, 24.35) -> (12.2238, 24.05)
  line L100 (12.2238, 24.05) -> (12.3, 24.05)
  line L101 (12.3, 24.05) -> (12.3, 24.35)
  line L102 (12.05, 24.35) -> (11.9738, 24.35)
  line L103 (11.9738, 24.35) -> (11.9738, 24.05)
  line L104 (11.9738, 24.05) -> (12.05, 24.05)
  line L105 (12.05, 24.05) -> (12.05, 24.35)
  line L106 (11.8, 24.35) -> (11.7238, 24.35)
  line L107 (11.7238, 24.35) -> (11.7238, 24.05)
  line L108 (11.7238, 24.05) -> (11.8, 24.05)
  line L109 (11.8, 24.05) -> (11.8, 24.35)
  line L110 (11.55, 24.35) -> (11.4738, 24.35)
  line L111 (11.4738, 24.35) -> (11.4738, 24.05)
  line L112 (11.4738, 24.05) -> (11.55, 24.05)
  line L113 (11.55, 24.05) -> (11.55, 24.35)
  line L114 (11.3, 24.35) -> (11.2238, 24.35)
  line L115 (11.2238, 24.35) -> (11.2238, 24.05)
  line L116 (11.2238, 24.05) -> (11.3, 24.05)
  line L117 (11.3, 24.05) -> (11.3, 24.35)
  line L118 (11.05, 24.35) -> (10.9738, 24.35)
  line L119 (10.9738, 24.35) -> (10.9738, 24.05)
  line L120 (10.9738, 24.05) -> (11.05, 24.05)
  line L121 (11.05, 24.05) -> (11.05, 24.35)
  line L122 (10.8, 24.35) -> (10.7238, 24.35)
  line L123 (10.7238, 24.35) -> (10.7238, 24.05)
  line L124 (10.7238, 24.05) -> (10.8, 24.05)
  line L125 (10.8, 24.05) -> (10.8, 24.35)
  line L126 (10.55, 24.35) -> (10.4738, 24.35)
  line L127 (10.4738, 24.35) -> (10.4738, 24.05)
  line L128 (10.4738, 24.05) -> (10.55, 24.05)
  line L129 (10.55, 24.05) -> (10.55, 24.35)
  line L130 (10.3, 24.35) -> (10.2238, 24.35)
  line L131 (10.2238, 24.35) -> (10.2238, 24.05)
  line L132 (10.2238, 24.05) -> (10.3, 24.05)
  line L133 (10.3, 24.05) -> (10.3, 24.35)
  line L134 (10.05, 24.35) -> (9.9738, 24.35)
  line L135 (9.9738, 24.35) -> (9.9738, 24.05)
  line L136 (9.9738, 24.05) -> (10.05, 24.05)
  line L137 (10.05, 24.05) -> (10.05, 24.35)
  line L138 (9.8, 24.35) -> (9.7238, 24.35)
  line L139 (9.7238, 24.35) -> (9.7238, 24.05)
  line L140 (9.7238, 24.05) -> (9.8, 24.05)
  line L141 (9.8, 24.05) -> (9.8, 24.35)
  line L142 (9.55, 24.35) -> (9.4738, 24.35)
  line L143 (9.4738, 24.35) -> (9.4738, 24.05)
  line L144 (9.4738, 24.05) -> (9.55, 24.05)
  line L145 (9.55, 24.05) -> (9.55, 24.35)
  line L146 (9.3, 24.35) -> (9.2238, 24.35)
  line L147 (9.2238, 24.35) -> (9.2238, 24.05)
  line L148 (9.2238, 24.05) -> (9.3, 24.05)
  line L149 (9.3, 24.05) -> (9.3, 24.35)
  line L150 (9.05, 24.35) -> (8.9738, 24.35)
  line L151 (8.9738, 24.35) -> (8.9738, 24.05)
  line L152 (8.9738, 24.05) -> (9.05, 24.05)
  line L153 (9.05, 24.05) -> (9.05, 24.35)
  line L154 (8.8, 24.35) -> (8.7238, 24.35)
  line L155 (8.7238, 24.35) -> (8.7238, 24.05)
  line L156 (8.7238, 24.05) -> (8.8, 24.05)
  line L157 (8.8, 24.05) -> (8.8, 24.35)
  line L158 (8.55, 24.35) -> (8.4738, 24.35)
  line L159 (8.4738, 24.35) -> (8.4738, 24.05)
  line L160 (8.4738, 24.05) -> (8.55, 24.05)
  line L161 (8.55, 24.05) -> (8.55, 24.35)
  line L162 (8.3, 24.35) -> (8.2238, 24.35)
  line L163 (8.2238, 24.35) -> (8.2238, 24.05)
  line L164 (8.2238, 24.05) -> (8.3, 24.05)
  line L165 (8.3, 24.05) -> (8.3, 24.35)
  line L166 (8.05, 24.35) -> (7.9738, 24.35)
  line L167 (7.9738, 24.35) -> (7.9738, 24.05)
  line L168 (7.9738, 24.05) -> (8.05, 24.05)
  line L169 (8.05, 24.05) -> (8.05, 24.35)
  line L170 (7.8, 24.35) -> (7.7238, 24.35)
  line L171 (7.7238, 24.35) -> (7.7238, 24.05)
  line L172 (7.7238, 24.05) -> (7.8, 24.05)
  line L173 (7.8, 24.05) -> (7.8, 24.35)
  line L174 (7.55, 24.35) -> (7.4738, 24.35)
  line L175 (7.4738, 24.35) -> (7.4738, 24.05)
  line L176 (7.4738, 24.05) -> (7.55, 24.05)
  line L177 (7.55, 24.05) -> (7.55, 24.35)
  line L178 (7.3, 24.35) -> (7.2238, 24.35)
  line L179 (7.2238, 24.35) -> (7.2238, 24.05)
  line L180 (7.2238, 24.05) -> (7.3, 24.05)
  line L181 (7.3, 24.05) -> (7.3, 24.35)
  line L182 (7.05, 24.35) -> (6.9738, 24.35)
  line L183 (6.9738, 24.35) -> (6.9738, 24.05)
  line L184 (6.9738, 24.05) -> (7.05, 24.05)
  line L185 (7.05, 24.05) -> (7.05, 24.35)
  line L186 (6.8, 24.35) -> (6.7238, 24.35)
  line L187 (6.7238, 24.35) -> (6.7238, 24.05)
  line L188 (6.7238, 24.05) -> (6.8, 24.05)
  line L189 (6.8, 24.05) -> (6.8, 24.35)
  line L190 (6.55, 24.35) -> (6.4738, 24.35)
  line L191 (6.4738, 24.35) -> (6.4738, 24.05)
  line L192 (6.4738, 24.05) -> (6.55, 24.05)
  line L193 (6.55, 24.05) -> (6.55, 24.35)
  line L194 (6.3, 24.35) -> (6.2238, 24.35)
  line L195 (6.2238, 24.35) -> (6.2238, 24.05)
  line L196 (6.2238, 24.05) -> (6.3, 24.05)
  line L197 (6.3, 24.05) -> (6.3, 24.35)
  line L198 (6.05, 24.35) -> (5.9738, 24.35)
  line L199 (5.9738, 24.35) -> (5.9738, 24.05)
  line L200 (5.9738, 24.05) -> (6.05, 24.05)
  line L201 (6.05, 24.05) -> (6.05, 24.35)
  line L202 (5.8, 24.35) -> (5.7238, 24.35)
  line L203 (5.7238, 24.35) -> (5.7238, 24.05)
  line L204 (5.7238, 24.05) -> (5.8, 24.05)
  line L205 (5.8, 24.05) -> (5.8, 24.35)
  line L206 (5.55, 24.35) -> (5.4738, 24.35)
  line L207 (5.4738, 24.35) -> (5.4738, 24.05)
  line L208 (5.4738, 24.05) -> (5.55, 24.05)
  line L209 (5.55, 24.05) -> (5.55, 24.35)
  line L210 (5.3, 24.35) -> (5.2238, 24.35)
  line L211 (5.2238, 24.35) -> (5.2238, 24.05)
  line L212 (5.2238, 24.05) -> (5.3, 24.05)
  line L213 (5.3, 24.05) -> (5.3, 24.35)
  line L214 (5.05, 24.35) -> (4.9738, 24.35)
  line L215 (4.9738, 24.35) -> (4.9738, 24.05)
  line L216 (4.9738, 24.05) -> (5.05, 24.05)
  line L217 (5.05, 24.05) -> (5.05, 24.35)
  line L218 (4.8, 24.35) -> (4.7238, 24.35)
  line L219 (4.7238, 24.35) -> (4.7238, 24.05)
  line L220 (4.7238, 24.05) -> (4.8, 24.05)
  line L221 (4.8, 24.05) -> (4.8, 24.35)
  line L222 (4.55, 24.35) -> (4.4738, 24.35)
  line L223 (4.4738, 24.35) -> (4.4738, 24.05)
  line L224 (4.4738, 24.05) -> (4.55, 24.05)
  line L225 (4.55, 24.05) -> (4.55, 24.35)
  line L226 (4.3, 24.35) -> (4.2238, 24.35)
  line L227 (4.2238, 24.35) -> (4.2238, 24.05)
  line L228 (4.2238, 24.05) -> (4.3, 24.05)
  line L229 (4.3, 24.05) -> (4.3, 24.35)
  line L230 (4.05, 24.35) -> (3.9738, 24.35)
  line L231 (3.9738, 24.35) -> (3.9738, 24.05)
  line L232 (3.9738, 24.05) -> (4.05, 24.05)
  line L233 (4.05, 24.05) -> (4.05, 24.35)
  line L234 (3.8, 24.35) -> (3.7238, 24.35)
  line L235 (3.7238, 24.35) -> (3.7238, 24.05)
  line L236 (3.7238, 24.05) -> (3.8, 24.05)
  line L237 (3.8, 24.05) -> (3.8, 24.35)
  line L238 (3.55, 24.35) -> (3.4738, 24.35)
  line L239 (3.4738, 24.35) -> (3.4738, 24.05)
  line L240 (3.4738, 24.05) -> (3.55, 24.05)
  line L241 (3.55, 24.05) -> (3.55, 24.35)
  line L242 (3.3, 24.35) -> (3.2238, 24.35)
  line L243 (3.2238, 24.35) -> (3.2238, 24.05)
  line L244 (3.2238, 24.05) -> (3.3, 24.05)
  line L245 (3.3, 24.05) -> (3.3, 24.35)
  line L246 (3.05, 24.35) -> (2.9738, 24.35)
  line L247 (2.9738, 24.35) -> (2.9738, 24.05)
  line L248 (2.9738, 24.05) -> (3.05, 24.05)
  line L249 (3.05, 24.05) -> (3.05, 24.35)
  line L250 (2.8, 24.35) -> (2.7238, 24.35)
  line L251 (2.7238, 24.35) -> (2.7238, 24.05)
  line L252 (2.7238, 24.05) -> (2.8, 24.05)
  line L253 (2.8, 24.05) -> (2.8, 24.35)
  line L254 (2.55, 24.35) -> (2.4738, 24.35)
  line L255 (2.4738, 24.35) -> (2.4738, 24.05)
  line L256 (2.4738, 24.05) -> (2.55, 24.05)
  line L257 (2.55, 24.05) -> (2.55, 24.35)
  line L258 (2.3, 24.35) -> (2.2238, 24.35)
  line L259 (2.2238, 24.35) -> (2.2238, 24.05)
  line L260 (2.2238, 24.05) -> (2.3, 24.05)
  line L261 (2.3, 24.05) -> (2.3, 24.35)
  line L262 (2.05, 24.35) -> (1.9738, 24.35)
  line L263 (1.9738, 24.35) -> (1.9738, 24.05)
  line L264 (1.9738, 24.05) -> (2.05, 24.05)
  line L265 (2.05, 24.05) -> (2.05, 24.35)
  line L266 (1.8, 24.35) -> (1.7238, 24.35)
  line L267 (1.7238, 24.35) -> (1.7238, 24.05)
  line L268 (1.7238, 24.05) -> (1.8, 24.05)
  line L269 (1.8, 24.05) -> (1.8, 24.35)
  line L270 (1.55, 24.35) -> (1.4738, 24.35)
  line L271 (1.4738, 24.35) -> (1.4738, 24.05)
  line L272 (1.4738, 24.05) -> (1.55, 24.05)
  line L273 (1.55, 24.05) -> (1.55, 24.35)
  line L274 (1.3, 24.35) -> (1.2238, 24.35)
  line L275 (1.2238, 24.35) -> (1.2238, 24.05)
  line L276 (1.2238, 24.05) -> (1.3, 24.05)
  line L277 (1.3, 24.05) -> (1.3, 24.35)
  line L278 (1.05, 24.35) -> (0.9738, 24.35)
  line L279 (0.9738, 24.35) -> (0.9738, 24.05)
  line L280 (0.9738, 24.05) -> (1.05, 24.05)
  line L281 (1.05, 24.05) -> (1.05, 24.35)
  line L282 (0.8, 24.35) -> (0.7238, 24.35)
  line L283 (0.7238, 24.35) -> (0.7238, 24.05)
  line L284 (0.7238, 24.05) -> (0.8, 24.05)
  line L285 (0.8, 24.05) -> (0.8, 24.35)
  line L286 (18.175, 23.9738) -> (18.0988, 23.9738)
  line L287 (18.0988, 23.9738) -> (18.0988, 23.6738)
  line L288 (18.0988, 23.6738) -> (18.175, 23.6738)
  line L289 (18.175, 23.6738) -> (18.175, 23.9738)
  line L290 (17.8488, 23.9738) -> (17.8488, 23.6738)
  line L291 (17.925, 23.9738) -> (17.8488, 23.9738)
  line L292 (17.8488, 23.6738) -> (17.925, 23.6738)
  line L293 (17.925, 23.6738) -> (17.925, 23.9738)
  line L294 (17.5988, 23.9738) -> (17.5988, 23.6738)
  line L295 (17.675, 23.9738) -> (17.5988, 23.9738)
  line L296 (17.5988, 23.6738) -> (17.675, 23.6738)
  line L297 (17.675, 23.6738) -> (17.675, 23.9738)
  line L298 (17.3488, 23.9738) -> (17.3488, 23.6738)
  line L299 (17.425, 23.9738) -> (17.3488, 23.9738)
  line L300 (17.3488, 23.6738) -> (17.425, 23.6738)
  line L301 (17.425, 23.6738) -> (17.425, 23.9738)
  line L302 (17.0988, 23.9738) -> (17.0988, 23.6738)
  line L303 (17.175, 23.9738) -> (17.0988, 23.9738)
  line L304 (17.0988, 23.6738) -> (17.175, 23.6738)
  line L305 (17.175, 23.6738) -> (17.175, 23.9738)
  line L306 (16.8488, 23.9738) -> (16.8488, 23.6738)
  line L307 (16.925, 23.9738) -> (16.8488, 23.9738)
  line L308 (16.8488, 23.6738) -> (16.925, 23.6738)
  line L309 (16.925, 23.6738) -> (16.925, 23.9738)
  line L310 (16.5988, 23.9738) -> (16.5988, 23.6738)
  line L311 (16.675, 23.9738) -> (16.5988, 23.9738)
  line L312 (16.5988, 23.6738) -> (16.675, 23.6738)
  line L313 (16.675, 23.6738) -> (16.675, 23.9738)
  line L314 (16.3488, 23.9738) -> (16.3488, 23.6738)
  line L315 (16.425, 23.9738) -> (16.3488, 23.9738)
  line L316 (16.3488, 23.6738) -> (16.425, 23.6738)
  line L317 (16.425, 23.6738) -> (16.425, 23.9738)
  line L318 (16.0988, 23.9738) -> (16.0988, 23.6738)
  line L319 (16.175, 23.9738) -> (16.0988, 23.9738)
  line L320 (16.0988, 23.6738) -> (16.175, 23.6738)
  line L321 (16.175, 23.6738) -> (16.175, 23.9738)
  line L322 (15.8488, 23.9738) -> (15.8488, 23.6738)
  line L323 (15.925, 23.9738) -> (15.8488, 23.9738)
  line L324 (15.8488, 23.6738) -> (15.925, 23.6738)
  line L325 (15.925, 23.6738) -> (15.925, 23.9738)
  line L326 (15.5988, 23.9738) -> (15.5988, 23.6738)
  line L327 (15.675, 23.9738) -> (15.5988, 23.9738)
  line L328 (15.5988, 23.6738) -> (15.675, 23.6738)
  line L329 (15.675, 23.6738) -> (15.675, 23.9738)
  line L330 (15.3488, 23.9738) -> (15.3488, 23.6738)
  line L331 (15.425, 23.9738) -> (15.3488, 23.9738)
  line L332 (15.3488, 23.6738) -> (15.425, 23.6738)
  line L333 (15.425, 23.6738) -> (15.425, 23.9738)
  line L334 (15.0988, 23.9738) -> (15.0988, 23.6738)
  line L335 (15.175, 23.9738) -> (15.0988, 23.9738)
  line L336 (15.0988, 23.6738) -> (15.175, 23.6738)
  line L337 (15.175, 23.6738) -> (15.175, 23.9738)
  line L338 (14.8488, 23.9738) -> (14.8488, 23.6738)
  line L339 (14.925, 23.9738) -> (14.8488, 23.9738)
  line L340 (14.8488, 23.6738) -> (14.925, 23.6738)
  line L341 (14.925, 23.6738) -> (14.925, 23.9738)
  line L342 (14.5988, 23.9738) -> (14.5988, 23.6738)
  line L343 (14.675, 23.9738) -> (14.5988, 23.9738)
  line L344 (14.5988, 23.6738) -> (14.675, 23.6738)
  line L345 (14.675, 23.6738) -> (14.675, 23.9738)
  line L346 (14.3488, 23.9738) -> (14.3488, 23.6738)
  line L347 (14.425, 23.9738) -> (14.3488, 23.9738)
  line L348 (14.3488, 23.6738) -> (14.425, 23.6738)
  line L349 (14.425, 23.6738) -> (14.425, 23.9738)
  line L350 (14.0988, 23.9738) -> (14.0988, 23.6738)
  line L351 (14.175, 23.9738) -> (14.0988, 23.9738)
  line L352 (14.0988, 23.6738) -> (14.175, 23.6738)
  line L353 (14.175, 23.6738) -> (14.175, 23.9738)
  line L354 (13.8488, 23.9738) -> (13.8488, 23.6738)
  line L355 (13.925, 23.9738) -> (13.8488, 23.9738)
  line L356 (13.8488, 23.6738) -> (13.925, 23.6738)
  line L357 (13.925, 23.6738) -> (13.925, 23.9738)
  line L358 (13.5988, 23.9738) -> (13.5988, 23.6738)
  line L359 (13.675, 23.9738) -> (13.5988, 23.9738)
  line L360 (13.5988, 23.6738) -> (13.675, 23.6738)
  line L361 (13.675, 23.6738) -> (13.675, 23.9738)
  line L362 (13.3488, 23.9738) -> (13.3488, 23.6738)
  line L363 (13.425, 23.9738) -> (13.3488, 23.9738)
  line L364 (13.3488, 23.6738) -> (13.425, 23.6738)
  line L365 (13.425, 23.6738) -> (13.425, 23.9738)
  line L366 (13.0988, 23.9738) -> (13.0988, 23.6738)
  line L367 (13.175, 23.9738) -> (13.0988, 23.9738)
  line L368 (13.0988, 23.6738) -> (13.175, 23.6738)
  line L369 (13.175, 23.6738) -> (13.175, 23.9738)
  line L370 (12.8488, 23.9738) -> (12.8488, 23.6738)
  line L371 (12.925, 23.9738) -> (12.8488, 23.9738)
  line L372 (12.8488, 23.6738) -> (12.925, 23.6738)
  line L373 (12.925, 23.6738) -> (12.925, 23.9738)
  line L374 (12.5988, 23.9738) -> (12.5988, 23.6738)
  line L375 (12.675, 23.9738) -> (12.5988, 23.9738)
  line L376 (12.5988, 23.6738) -> (12.675, 23.6738)
  line L377 (12.675, 23.6738) -> (12.675, 23.9738)
  line L378 (12.3488, 23.9738) -> (12.3488, 23.6738)
  line L379 (12.425, 23.9738) -> (12.3488, 23.9738)
  line L380 (12.3488, 23.6738) -> (12.425, 23.6738)
  line L381 (12.425, 23.6738) -> (12.425, 23.9738)
  line L382 (12.0988, 23.9738) -> (12.0988, 23.6738)
  line L383 (12.175, 23.9738) -> (12.0988, 23.9738)
  line L384 (12.0988, 23.6738) -> (12.175, 23.6738)
  line L385 (12.175, 23.6738) -> (12.175, 23.9738)
  line L386 (11.8488, 23.9738) -> (11.8488, 23.6738)
  line L387 (11.925, 23.9738) -> (11.8488, 23.9738)
  line L388 (11.8488, 23.6738) -> (11.925, 23.6738)
  line L389 (11.925, 23.6738) -> (11.925, 23.9738)
  line L390 (11.5988, 23.9738) -> (11.5988, 23.6738)
  line L391 (11.675, 23.9738) -> (11.5988, 23.9738)
  line L392 (11.5988, 23.6738) -> (11.675, 23.6738)
  line L393 (11.675, 23.6738) -> (11.675, 23.9738)
  line L394 (11.3488, 23.9738) -> (11.3488, 23.6738)
  line L395 (11.425, 23.9738) -> (11.3488, 23.9738)
  line L396 (11.3488, 23.6738) -> (11.425, 23.6738)
  line L397 (11.425, 23.6738) -> (11.425, 23.9738)
  line L398 (11.0988, 23.9738) -> (11.0988, 23.6738)
  line L399 (11.175, 23.9738) -> (11.0988, 23.9738)
  line L400 (11.0988, 23.6738) -> (11.175, 23.6738)
  line L401 (11.175, 23.6738) -> (11.175, 23.9738)
  line L402 (10.8488, 23.9738) -> (10.8488, 23.6738)
  line L403 (10.925, 23.9738) -> (10.8488, 23.9738)
  line L404 (10.8488, 23.6738) -> (10.925, 23.6738)
  line L405 (10.925, 23.6738) -> (10.925, 23.9738)
  line L406 (10.5988, 23.9738) -> (10.5988, 23.6738)
  line L407 (10.675, 23.9738) -> (10.5988, 23.9738)
  line L408 (10.5988, 23.6738) -> (10.675, 23.6738)
  line L409 (10.675, 23.6738) -> (10.675, 23.9738)
  line L410 (10.3488, 23.9738) -> (10.3488, 23.6738)
  line L411 (10.425, 23.9738) -> (10.3488, 23.9738)
  line L412 (10.3488, 23.6738) -> (10.425, 23.6738)